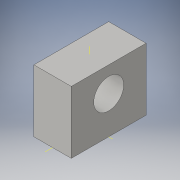
# Autodesk Inventor part: derived_drive_handle
Saved by Autodesk Inventor 2016 (Build 200138000, 138)
## iProperties
Created: 2016-07-02
Part Number: derived_drive_handle
Material: Generic
Document SubType Name: Modeling
Designer: GentnerLab
Density: 1 g/cm^3
Appearance: Default
Author: GentnerLab
Autodesk Inventor part; units mm, degrees
ref_plane "YZ Plane" through (0, 0, 0) normal (1, 0, 0) x (0, 1, 0)
ref_plane "XZ Plane" through (0, 0, 0) normal (0, 1, 0) x (-1, 0, 0)
ref_plane "XY Plane" through (0, 0, 0) normal (0, 0, 1) x (1, 0, 0)
sketch "base+body" plane through (0, 0, 0) normal (0, 1, 0) x (-1, 0, 0)
  circle A0 centre (0, 0) radius 2
  line L0 (-0.75, 1.5) -> (0.75, 1.5)
  line L1 (0.75, 1.5) -> (0.75, -1.5)
  line L2 (0.75, -1.5) -> (-0.75, -1.5)
  line L3 (-0.75, -1.5) -> (-0.75, 1.5)
  line L4 (-0.75, 1.5) -> (0.75, -1.5) construction
  line L5 (0.75, 1.5) -> (-0.75, -1.5) construction
  line L6 (-1.5, 0.525) -> (1.5, 0.525)
  line L7 (1.5, 0.525) -> (1.5, -0.525)
  line L8 (1.5, -0.525) -> (-1.5, -0.525)
  line L9 (-1.5, -0.525) -> (-1.5, 0.525)
  line L10 (-1.5, 0.525) -> (1.5, -0.525) construction
  line L11 (1.5, 0.525) -> (-1.5, -0.525) construction
  line L12 (0, 0.525) -> (2, 0.525)
  line L13 (2, 0.525) -> (2, -0.525)
  line L14 (2, -0.525) -> (0, -0.525)
  line L15 (0, -0.525) -> (0, 0.525)
  dimension "d0" = 4
  dimension "d1" = 3
  dimension "d2" = 1.5
  dimension "d3" = 1.05
  dimension "d4" = 3
  dimension "d5" = 1.05
  dimension "d6" = 2
  constraints: 32 end point, 6 parallel, 5 midpoint, 3 horizontal, 3 perpendicular, 1 centre point, 1 coincident
  measures "d0" diameter of A0
  measures "d1" distance between parallel lines of L0 L2
  measures "d2" distance between parallel lines of L3 L1
  measures "d3" distance between parallel lines of L8 L6
  measures "d4" distance between parallel lines of L9 L7
  measures "d5" distance between parallel lines of L14 L12
  measures "d6" distance from line of A0.centre L13
extrude "Extrusion1" add sketch "base+body" along normal blind 2.5 contours L6 L3 L0 L1 | L1 L8 L15 L6 | L1 L2 L3 L8 | L15 L8 L3 L6
sketch "Sketch3" plane through (0.75, 0, 1.5) normal (1, 0, 0) x (0, 0, -1)
  line L0 (3, 0) -> (3, 2.5) projected
  line L1 (0, 0) -> (0, 2.5) projected
  point P0 (1.5, 0)
  point P1 (1.5, 1.5)
  dimension "d9" = 1.5
  dimension "d10" = 3
  dimension "d11" = 2.5
  dimension "d12" = 1.5
  measures "d9" distance from line of L0 point (1.5, 1.5)
  measures "d10" distance between parallel lines of L0 L1
  measures "d11" distance of L0.start L0.end
  measures "d12" distance of point (1.5, 0) point (1.5, 1.5)
hole "Hole1" at (0.75, 1.5, 0) direction (-1, 0, 0) diameter 1.2 end through all
equation "\"d3\" = 0.7 * d2"
equation "\"d4\" = d1"
equation "\"d5\" = d3"
equation "\"d6\" = 0.5 * d0"
equation "\"d9\" = 0.5 * d10"
body "Solid1"
